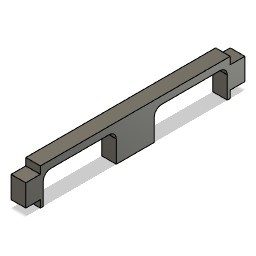
Стойки под контейнеры v3 (Autodesk Fusion 360 design; units mm, degrees)
Autodesk Fusion 360 part; units mm, degrees
sketch "Sketch1" plane through (0, 0, 0) normal (1, 0, 0) x (0, 0, -1)
  line L0 (0, 0) -> (-150, 0)
  line L1 (-150, 0) -> (-150, 25)
  line L2 (-150, 25) -> (0, 25)
  line L3 (0, 25) -> (0, 0)
  line L4 (-10, 0) -> (-140, 0)
  line L5 (-140, 0) -> (-140, 25)
  line L6 (-140, 25) -> (-10, 25)
  line L7 (-10, 25) -> (-10, 0)
  line L8 (-140, 20) -> (-150, 20)
  line L9 (-150, 20) -> (-150, 5)
  line L10 (-150, 5) -> (-140, 5)
  line L11 (-140, 5) -> (-140, 20)
  line L12 (-10, 5) -> (0, 5)
  line L13 (0, 5) -> (0, 20)
  line L14 (0, 20) -> (-10, 20)
  line L15 (-10, 20) -> (-10, 5)
  dimension "d1" = 150
  dimension "d2" = 25
  dimension "d3" = 130
  dimension "d4" = 25
  constraint horizontal L0
  constraint vertical L1
  constraint horizontal L2
  constraint vertical L3
  constraint coincident L0.start L3.end
  constraint horizontal L4
  constraint vertical L5
  constraint horizontal L6
  constraint vertical L7
  constraint coincident L0 L4.start
  constraint horizontal L8
  constraint vertical L9
  constraint horizontal L10
  constraint vertical L11
  constraint coincident L1 L9.end
  constraint coincident L5 L8.start
  constraint horizontal L12
  constraint vertical L13
  constraint horizontal L14
  constraint vertical L15
  constraint coincident L3 L13.end
  constraint coincident L7 L12.start
  measures "d1" distance of L0.start L0.end
  measures "d2" distance of L0.start L2.end
  measures "d3" distance of L4.start L4.end
  measures "d4" distance of L4.start L6.end
extrude "Extrude1" add sketch "Sketch1" along normal blind 10 contours L0 L2 L4 L5 L6 L7 L11 L15 | L3 L7 L12 L13 L14 L15 | L1 L5 L8 L9 L10 L11
sketch "Sketch2" plane through (0, 0, 0) normal (0, -1, 0) x (1, 0, 0)
  line L0 (0, 140) -> (0, 10)
  line L1 (0, 10) -> (10, 10)
  line L2 (10, 10) -> (10, 140)
  line L3 (10, 140) -> (0, 140)
  line L4 (0, 140) -> (10, 140)
  line L5 (10, 140) -> (10, 88)
  line L6 (10, 88) -> (0, 88)
  line L7 (0, 88) -> (0, 140)
  line L8 (0, 10) -> (10, 10)
  line L9 (10, 10) -> (10, 62)
  line L10 (10, 62) -> (0, 62)
  line L11 (0, 62) -> (0, 10)
  line L12 (0, 140) -> (10, 140)
  line L13 (10, 140) -> (10, 138)
  line L14 (10, 138) -> (0, 138)
  line L15 (0, 138) -> (0, 140)
  line L16 (0, 10) -> (10, 10)
  line L17 (10, 10) -> (10, 12)
  line L18 (10, 12) -> (0, 12)
  line L19 (0, 12) -> (0, 10)
  dimension "d7" = 52
  dimension "d8" = 52
  dimension "d9" = 2
  constraint horizontal L4
  constraint vertical L5
  constraint horizontal L6
  constraint vertical L7
  constraint coincident L0.start L3.end
  constraint horizontal L8
  constraint vertical L9
  constraint horizontal L10
  constraint vertical L11
  constraint coincident L0.end L1.start
  constraint horizontal L12
  constraint vertical L13
  constraint horizontal L14
  constraint vertical L15
  constraint coincident L2 L13.end
  constraint coincident L5 L13.end
  constraint horizontal L16
  constraint vertical L17
  constraint horizontal L18
  constraint vertical L19
  measures "d7" distance of L0.start L6.end
  measures "d8" distance of L0.end L10.end
  measures "d9" distance of L0.end L18.end
extrude "Extrude2" cut sketch "Sketch2" against normal blind 20 contours L0 L2 L5 L6 L7 L14 | L0 L2 L9 L10 L11 L18
fillet "Fillet1" radius 5 4 edges at (5, 20, 138) (5, 20, 88) (5, 20, 62) (5, 20, 12)
